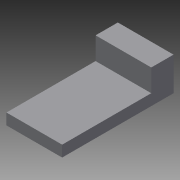
# Autodesk Inventor part: hook
Saved by Autodesk Inventor 2015 (Build 190159000, 159)
## iProperties
Created: 2015-01-07
Part Number: hook
Material: Generic
Document SubType Name: Modeling
Designer: harrykuperstein
Density: 1 g/cm^3
Appearance: Default
Author: harrykuperstein
Autodesk Inventor part; units mm, degrees
ref_plane "YZ Plane" through (0, 0, 0) normal (1, 0, 0) x (0, 1, 0)
ref_plane "XZ Plane" through (0, 0, 0) normal (0, 1, 0) x (-1, 0, 0)
ref_plane "XY Plane" through (0, 0, 0) normal (0, 0, 1) x (1, 0, 0)
sketch "Sketch1" plane through (0, 0, 0) normal (0, 1, 0) x (-1, 0, 0)
  line L0 (0, 0) -> (63.5, 0)
  line L1 (63.5, 0) -> (63.5, 127)
  line L2 (63.5, 127) -> (0, 127)
  line L3 (0, 127) -> (0, 0)
  dimension "d0" = 63.5
  dimension "d1" = 127
  constraints: 8 end point, 2 parallel, 1 horizontal, 1 perpendicular
  measures "d0" distance of L1.end L2.end
  measures "d1" distance of L2.end L0.start
extrude "Extrusion1" add sketch "Sketch1" along normal blind 12.7
sketch "Sketch2" plane through (0, 12.7, 0) normal (0, 1, 0) x (1, 0, 0)
  line L0 (0, 0) -> (0, -25.4)
  line L1 (0, -127) -> (0, 0) projected
  line L2 (0, 0) -> (-63.5, 0)
  line L3 (0, 0) -> (-63.5, 0) projected
  line L4 (-63.5, 0) -> (-63.5, -25.4)
  line L5 (-63.5, 0) -> (-63.5, -127) projected
  line L6 (-63.5, -25.4) -> (0, -25.4)
  dimension "d4" = 25.4
  constraints: 8 end point, 2 point on line, 1 collinear, 1 perpendicular
  measures "d4" distance of L0.start L0.end
extrude "Extrusion2" add sketch "Sketch2" along normal blind 25.4
body "Solid1"
